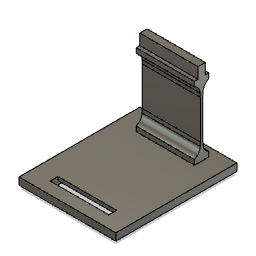
flexure thick v1 (Autodesk Fusion 360 design; units mm, degrees)
Autodesk Fusion 360 part; units mm, degrees
sketch "Sketch1" plane through (0, 0, 0) normal (1, 0, 0) x (0, 0, -1)
  line L0 (0, 0) -> (3, 0)
  line L1 (3, 0) -> (3, -4.5)
  line L2 (3, -4.5) -> (0, -4.5)
  line L3 (0, -4.5) -> (0, 0)
  line L4 (3, 0) -> (4.5, 0)
  line L5 (1.5, 0) -> (1.5, 16.3106) construction
  line L6 (-3.4591, 15) -> (5.8046, 15) construction
  line L7 (2, 15) -> (2, 7)
  line L8 (2, 7) -> (2.2, 3.005)
  line L9 (4.5, 0) -> (4.5, 2)
  line L10 (4.5, 2) -> (2.2, 3.005)
  line L11 (0, 0) -> (-1.5, 0)
  line L12 (-1.5, 0) -> (-1.5, 2)
  line L13 (-1.5, 2) -> (0.8, 3.005)
  line L14 (1, 7) -> (0.8, 3.005)
  line L15 (1, 15) -> (1, 7)
  line L16 (3, 30) -> (4.5, 30)
  line L17 (1, 23) -> (0.8, 26.995)
  line L18 (2, 23) -> (2.2, 26.995)
  line L19 (1, 15) -> (1, 23)
  line L20 (4.5, 30) -> (4.5, 28)
  line L21 (2, 15) -> (2, 23)
  line L22 (3, 30) -> (3, 34.5)
  line L23 (-1.5, 28) -> (0.8, 26.995)
  line L24 (0, 34.5) -> (0, 30)
  line L25 (3, 34.5) -> (0, 34.5)
  line L26 (0, 30) -> (-1.5, 30)
  line L27 (-1.5, 30) -> (-1.5, 28)
  line L28 (0, 30) -> (3, 30)
  line L29 (4.5, 28) -> (2.2, 26.995)
  point P0 (0, 30)
  point P1 (1.5, 30)
  dimension "d1" = 3
  dimension "d2" = 4.5
  dimension "d3" = 1.5
  dimension "d5" = 15
  dimension "d6" = 8
  dimension "d7" = 4
  dimension "d8" = 0.5
  dimension "d9" = 0.7
  dimension "d10" = 2
  constraint horizontal L0
  constraint vertical L1
  constraint horizontal L2
  constraint vertical L3
  constraint coincident L0.start L3.end
  constraint perpendicular L1 L4
  constraint midpoint L0 L5.start
  constraint perpendicular L0 L5
  constraint horizontal L6
  constraint coincident L6 L7.start
  constraint perpendicular L6 L7
  constraint perpendicular L4 L9
  constraint symmetric L0.end L5 L0.start
  constraint symmetric L4.end L5 L11.end
  constraint symmetric L5 L7.start L15.start
  constraint symmetric L5 L7.end L14.start
  constraint symmetric L5 L8.end L13.end
  constraint symmetric L5 L9.end L12.end
  constraint symmetric L0.start L6 L24.end
  constraint symmetric L0.start L6 P0
  constraint symmetric L0.end L6 L16.start
  constraint symmetric L1.end L6 L22.end
  constraint symmetric L2.end L6 L24.start
  constraint symmetric L4.end L6 L16.end
  constraint symmetric L5.start L6 P1
  constraint symmetric L6 L7.start L21.start
  constraint symmetric L6 L7.end L18.start
  constraint symmetric L6 L8.end L18.end
  constraint symmetric L6 L9.end L20.end
  constraint symmetric L6 L0.start P0
  constraint symmetric L6 L11.end L26.end
  constraint symmetric L6 L12.end L23.start
  constraint symmetric L6 L13.end L17.end
  constraint symmetric L6 L14.start L17.start
  constraint symmetric L6 L15.start L19.start
  measures "d1" distance of L0.start L0.end
  measures "d2" distance of L0.start L2.end
  measures "d3" distance of L0.end L4.end
  measures "d5" distance of L4 L6
  measures "d6" distance of L7.start L7.end
  measures "d7" distance of L7.end L8.end
  measures "d8" distance of L5 L7
  measures "d9" distance of L5 L8.end
  measures "d10" distance of L4.end L9.end
extrude "Extrude1" add sketch "Sketch1" along normal mid plane 24 makes body 1
sketch "Sketch2" plane through (0, 0, 0) normal (0, 1, 0) x (1, 0, 0)
  line L0 (-12, 0) -> (12, 0)
  line L1 (12, 0) -> (12, 3)
  line L2 (12, 3) -> (-12, 3)
  line L3 (-12, 3) -> (-12, 0)
  line L4 (12.1, 3.1) -> (-12.1, 3.1)
  line L5 (-12.1, 3.1) -> (-12.1, -0.1)
  line L6 (-12.1, -0.1) -> (12.1, -0.1)
  line L7 (12.1, -0.1) -> (12.1, 3.1)
  line L8 (0, 0) -> (0, -36.4952) construction
  line L9 (20, 8.1) -> (-20, 8.1)
  line L10 (-20, 8.1) -> (-20, -41.9)
  line L11 (-20, -41.9) -> (20, -41.9)
  line L12 (20, -41.9) -> (20, 8.1)
  line L13 (20, 8.1) -> (-20, -41.9) construction
  line L14 (-20, 8.1) -> (20, -41.9) construction
  line L15 (0, -16.9) -> (-15.1957, -16.9) construction
  line L16 (-12.1, -33.7) -> (12.1, -33.7)
  line L17 (12.1, -33.7) -> (12.1, -36.9)
  line L18 (12.1, -36.9) -> (-12.1, -36.9)
  line L19 (-12.1, -36.9) -> (-12.1, -33.7)
  point P0 (0, -16.9)
  dimension "d13" = 0.1
  dimension "d14" = 40
  dimension "d15" = 50
  dimension "d16" = 5
  constraint coincident L8.start origin
  constraint perpendicular L6 L8
  constraint horizontal L9
  constraint perpendicular L9 L10
  constraint parallel L9 L11
  constraint parallel L10 L12
  constraint coincident L13 P0
  constraint coincident L14 P0
  constraint coincident L8 P0
  constraint coincident P0 L15.start
  constraint perpendicular L8 L15
  constraint symmetric L4.start L15 L17.end
  constraint symmetric L4.end L15 L18.end
  constraint symmetric L5.end L15 L16.start
  constraint symmetric L6.end L15 L16.end
  measures "d14" distance of L10.end L11.end
  measures "d15" distance of L9.end L10.end
  measures "d16" distance of L4 L9
extrude "Extrude2" add sketch "Sketch2" against normal blind 3 separate body contours L9 L10 L11 L12 makes body 2
chamfer "Chamfer1" distance 1.5 angle 45 4 edges at (0, -3, -3.1) (0, -3, 0.1) (0, -3, 33.7) (0, -3, 36.9) on bodies 2
fillet "Fillet1" radius 4 4 edges at (0, 3.005, -0.8) (0, 3.005, -2.2) (0, 26.995, -0.8) (0, 26.995, -2.2) on bodies 1
named bodies: "flexure flex", "flexure plate"
